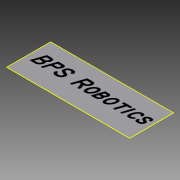
# Autodesk Inventor part: banner2
Saved by Autodesk Inventor 2014 (Build 180170000, 170)
## iProperties
Created: 2015-04-10
Part Number: banner2
Material: Generic
Document SubType Name: Modeling
Designer: Gus
Density: 1 g/cm^3
Appearance: Default
Author: Gus
Autodesk Inventor part; units mm, degrees
ref_plane "YZ Plane" through (0, 0, 0) normal (1, 0, 0) x (0, 1, 0)
ref_plane "XZ Plane" through (0, 0, 0) normal (0, 1, 0) x (-1, 0, 0)
ref_plane "XY Plane" through (0, 0, 0) normal (0, 0, 1) x (1, 0, 0)
sketch "Sketch1" plane through (0, 0, 0) normal (0, 1, 0) x (-1, 0, 0)
  line L0 (0, 0) -> (2133.6, 0)
  line L1 (2133.6, 0) -> (2133.6, 762)
  line L2 (2133.6, 762) -> (0, 762)
  line L3 (0, 762) -> (0, 0)
  dimension "d0" = 2133.6
  dimension "d1" = 762
  constraints: 8 end point, 2 parallel, 1 horizontal, 1 perpendicular
  measures "d0" distance of L2.end L1.end
  measures "d1" distance of L1.end L0.end
extrude "Extrusion1" add sketch "Sketch1" along normal blind 2.54
sketch "Sketch2" plane through (0, 2.54, 0) normal (0, 1, 0) x (1, 0, 0)
  line L0 (0, 0) -> (-2133.6, 0) projected
  line L1 (-2133.6, 0) -> (-2133.6, -762) projected
  line L2 (-2133.6, -762) -> (0, -762) projected
  line L3 (0, -762) -> (0, 0) projected
  line L4 (-2053.8257, -227.8408) -> (135.5229, -227.8408) construction
  line L5 (135.5229, -227.8408) -> (135.5229, -488.7997) construction
  line L6 (135.5229, -488.7997) -> (-2053.8257, -488.7997) construction
  line L7 (-2053.8257, -488.7997) -> (-2053.8257, -227.8408) construction
  constraints: 2 other
body "Solid1"
